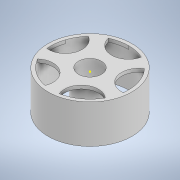
# Autodesk Inventor part: WheelGBR
Saved by Autodesk Inventor 2020.1 (Build 241239000, 239)
## iProperties
Created: 2020-03-09
Part Number: WheelGBR
Material: Generic
Document SubType Name: Modeling
Designer: super
Density: 1 g/cm^3
Appearance: Default
Author: super
Autodesk Inventor part; units mm, degrees
ref_plane "YZ Plane" through (0, 0, 0) normal (1, 0, 0) x (0, 1, 0)
ref_plane "XZ Plane" through (0, 0, 0) normal (0, 1, 0) x (-1, 0, 0)
ref_plane "XY Plane" through (0, 0, 0) normal (0, 0, 1) x (1, 0, 0)
sketch "Sketch1" plane through (0, 0, 0) normal (0, 1, 0) x (-1, 0, 0)
  circle A0 centre (0, 0) radius 5.588
  circle A1 centre (0, 0) radius 4.318
  circle A2 centre (0, 0) radius 14.478
  circle A3 centre (0, 0) radius 15.748
  dimension "d0" = 11.176
  dimension "d1" = 8.636
  dimension "d2" = 28.956
  dimension "d3" = 31.496
  constraints: 4 centre point, 4 coincident
  measures "d0" diameter of A0
  measures "d1" diameter of A1
  measures "d2" diameter of A2
  measures "d3" diameter of A3
extrude "Extrusion1" add sketch "Sketch1" along normal blind 14.478
sketch "Sketch2" plane through (0, 14.478, 0) normal (0, 1, 0) x (1, 0, 0)
  circle A0 centre (0, 0) radius 14.478
  circle A1 centre (0, 0) radius 5.588
  constraints: 2 centre point, 2 coincident
extrude "Extrusion2" add sketch "Sketch2" against normal blind 1.27
sketch "Sketch3" plane through (0, 13.208, 0) normal (0, -1, 0) x (1, 0, 0)
  circle A0 centre (0, 0) radius 14.478
  arc A1 (6.197477, -13.094605) -> (-6.195427, -13.085456) centre (0, -14.478) ccw
  arc A2 (-6.195427, -13.085456) -> (6.197477, -13.094605) centre (0.010723, 0.047707) ccw
  circle A3 centre (0, 0) radius 14.478
  circle A4 centre (0, 0) radius 5.588
  arc A5 (14.368835, 1.847695) -> (10.530516, -9.93583) centre (13.769396, -4.473948) ccw
  arc A6 (10.530516, -9.93583) -> (14.368835, 1.847695) centre (-0.042059, 0.024941) ccw
  arc A7 (2.682952, 14.236543) -> (12.703644, 6.944775) centre (8.509955, 11.712948) ccw
  arc A8 (12.703644, 6.944775) -> (2.682952, 14.236543) centre (-0.036717, -0.032293) ccw
  arc A9 (-12.71068, 6.950972) -> (-2.679232, 14.227937) centre (-8.509955, 11.712948) ccw
  arc A10 (-2.679232, 14.227937) -> (-12.71068, 6.950972) centre (0.019366, -0.044899) ccw
  arc A11 (-10.538584, -9.940606) -> (-14.359501, 1.848573) centre (-13.769396, -4.473948) ccw
  arc A12 (-14.359501, 1.848573) -> (-10.538584, -9.940606) centre (0.048686, 0.004544) ccw
  point P0 (-8.509955, 11.712948)
  point P1 (-12.703644, 6.944775)
  point P2 (8.509955, 11.712948)
  point P3 (2.679232, 14.227937)
  point P4 (-10.530516, -9.93583)
  point P5 (6.195427, -13.085456)
  point P6 (13.769396, -4.473948)
  point P7 (14.359501, 1.848573)
  dimension "d8" = 6.35
  dimension "d11" = 360
  constraints: 27 point on circle, 10 centre point, 31 other
  measures "d8" radius of A1
sketch "Sketch3 outline for Extrusion3" plane through (0, 13.208, 0) normal (0, -1, 0) x (1, 0, 0)
  arc A0 (-2.679232, 14.227937) -> (-8.509955, 11.712948) centre (0.019366, -0.044899) ccw
  arc A1 (-12.703644, 6.944775) -> (-2.679232, 14.227937) centre (-8.509955, 11.712948) ccw
  arc A2 (-8.509955, 11.712948) -> (-12.703644, 6.944775) centre (0, 0) ccw
  arc A3 (12.703644, 6.944775) -> (8.509955, 11.712948) centre (-0.036717, -0.032293) ccw
  arc A4 (2.679232, 14.227937) -> (12.703644, 6.944775) centre (8.509955, 11.712948) ccw
  arc A5 (8.509955, 11.712948) -> (2.679232, 14.227937) centre (0, 0) ccw
  arc A6 (-14.359501, 1.848573) -> (-13.769396, -4.473948) centre (0.048686, 0.004544) ccw
  arc A7 (-10.530516, -9.93583) -> (-14.359501, 1.848573) centre (-13.769396, -4.473948) ccw
  arc A8 (-13.769396, -4.473948) -> (-10.530516, -9.93583) centre (0, 0) ccw
  arc A9 (-6.195427, -13.085456) -> (0, -14.478) centre (0.010723, 0.047707) ccw
  arc A10 (6.195427, -13.085456) -> (-6.195427, -13.085456) centre (0, -14.478) ccw
  arc A11 (0, -14.478) -> (6.195427, -13.085456) centre (0, 0) ccw
  arc A12 (10.530516, -9.93583) -> (13.769396, -4.473948) centre (-0.042059, 0.024941) ccw
  arc A13 (14.359501, 1.848573) -> (10.530516, -9.93583) centre (13.769396, -4.473948) ccw
  arc A14 (13.769396, -4.473948) -> (14.359501, 1.848573) centre (0, 0) ccw
extrude "Extrusion3" cut sketch "Sketch3 outline for Extrusion3" against normal blind 25.4
sketch "Sketch4" plane through (0, 13.208, 0) normal (0, -1, 0) x (1, 0, 0)
  point P0 (0, 0)
body "Solid1"
